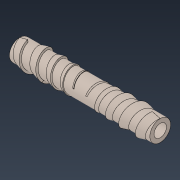
# Autodesk Inventor part: Dribblerschnecke v2
Saved by Autodesk Inventor 2022.3 (Build 263350000, 350)
## iProperties
Part Number: Dribblerschnecke v2
Material: Gummi, Silikon
Document SubType Name: Modeling
Designer: rYan
Mass: 5.52126 g
Surface Area: 49.6074 cm^2
Volume: 4.41701 cm^3
Density: 1.25 g/cm^3
Appearance: Gummi - Schwarz(3)
Author: rYan
Autodesk Inventor part; units mm, degrees
ref_plane "YZ Plane" through (0, 0, 0) normal (1, 0, 0) x (0, 1, 0)
ref_plane "XZ Plane" through (0, 0, 0) normal (0, 1, 0) x (-1, 0, 0)
ref_plane "XY Plane" through (0, 0, 0) normal (0, 0, 1) x (1, 0, 0)
sketch "Skizze1" plane through (0, 0, 0) normal (1, 0, 0) x (0, 1, 0)
  circle A0 centre (0, 0) radius 3
  circle A1 centre (0, 0) radius 5
  dimension "d0" = 6
  dimension "d1" = 10
  constraints: 2 centre point, 2 coincident
  measures "d0" diameter of A0
  measures "d1" diameter of A1
extrude "Extrusion1" add sketch "Skizze1" along normal blind 33.7
sketch "Skizze3" plane through (0, 0, 0) normal (0, 1, 0) x (-1, 0, 0)
  line L0 (-33.7, 5) -> (-29.7, 5)
  line L1 (-29.7, 5) -> (-29.8763, 6)
  line L2 (-29.8763, 6) -> (-33.7, 5)
  line L3 (-33.7, 5) -> (-33.7, -5) construction
  line L4 (0, -5) -> (0, 5) construction
  line L5 (-36.7, 5) -> (-36.8763, 6) construction
  circle A0 centre (-33.6009, 27.249) radius 21.5 construction
  line L6 (-28.161, 6.4486) -> (-33.6009, 27.249) construction
  line L7 (-29.8763, 6) -> (-36.8763, 6) construction
  point P0 (0, 0)
  dimension "d98" = 43
  dimension "d16" = 4
  dimension "d17" = 80
  dimension "d18" = 1
  dimension "d96" = 7
  dimension "d126" = 14.656
  constraints: 12 end point, 2 horizontal, 2 point on line, 1 coincident, 1 parallel, 1 perpendicular, 4 other
  measures "d16" distance of L0.start L0.end
  measures "d17" angle of L1 L0
  measures "d18" distance from line of L0 L1.end
  measures "d96" distance of L5.start L0.end
  measures "d126" angle of L0 L2
coil "Spirale1" sketch "Skizze3" operation add axis through (-10, 0, 0) along (-1, 0, 0) pitch 8 turns 1.375 hand left
sketch "Skizze20" plane through (18.7, -3.5355, -3.5355) normal (0, 0.7071068, -0.7071068) x (1, 0, 0)
  line L0 (4, 0) -> (0, 0) projected
  line L1 (4, 0) -> (0.1763, 1) projected
  line L2 (0.1763, 1) -> (0, 0) projected
  point P0 (-18.7, -5)
coil "Spirale3" sketch "Skizze20" operation add axis through (-10, 0, 0) along (-1, 0, 0) pitch 6.5 turns 1.230769 hand left taper -3
sketch "Skizze24" plane through (10.7739, 3.0836, -3.9359) normal (0, 0.7871835, 0.6167189) x (1, 0, 0)
  line L0 (2.323, 0) -> (0, 0) projected
  line L1 (2.323, 0) -> (0.1024, 0.5807) projected
  line L2 (0.1024, 0.5807) -> (0, 0) projected
  point P0 (-10.7739, -5)
coil "Spirale4" sketch "Skizze24" operation add axis through (-10, 0, 0) along (-1, 0, 0) pitch 5 turns 1.6 hand left taper -3
mirror "Spiegeln2" about plane through (0, 0, 0) normal (1, 0, 0) of "Extrusion1", "Spirale1", "Spirale3", "Spirale4"
sketch "Skizze25" plane through (2.8479, -4.8082, 1.3717) normal (0, -0.2743466, -0.9616309) x (1, 0, 0)
  circle A0 centre (-2.8479, 21.4682) radius 21.5
  circle A1 centre (1.449, 21.6145) radius 21.5
  circle A2 centre (13.3899, 22.0495) radius 21.5
  point P0 (-2.8479, -5)
  point P1 (-5.7242, 0.1615)
  point P2 (0.0285, 0.1615)
  dimension "d163" = 43
  dimension "d162" = 43
  dimension "d164" = 43
  constraints: 2 centre point, 2 point on circle, 3 other
  measures "d162" diameter of A0
  measures "d164" diameter of A2
